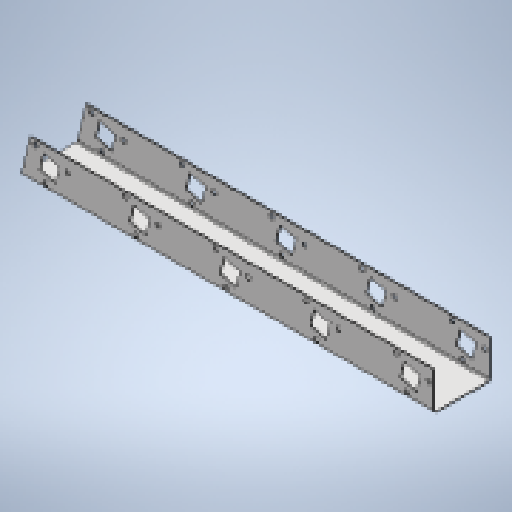
# Autodesk Inventor part: MNT-CDF-501 box
Saved by Autodesk Inventor 2025.1 (Build 291241020, 241B)
## iProperties
Created: 2025-01-13
Part Number: MNT-CDF-501 box
Material: Stainless Steel
Description: DIE16(5)|\ 90°|corrY -___°|X_____|bom___
Document SubType Name: Sheet Metal
Designer: user
Stock Number: МОО 305 шпангоут борт
Mass: 1762.25 g
Surface Area: 2283.33 cm^2
Volume: 220.281 cm^3
Density: 8 g/cm^3
Sheet Metal Rule: AISI304 2mm Die16
Sheet Metal Width: 0.000 mm
Sheet Metal Length: 0.000 mm
Sheet Metal Area: 0.000 mm^2
Appearance: Default
БОРТ_стрингер_3_высота: 63.000 mm
БОРТ_стрингер_4_высота: 48.000 mm
БОРТ_стрингер_5_высота: 54.000 mm
БОРТ_стрингер_6_высота: 81.000 mm
РЕБРА_глубина_паза: 28.000 mm
РЕБРА_вырез_на_полке: 5,000 mm
РЕБРА_полка: 20,000 mm
Author: user
Autodesk Inventor part; units mm, degrees
ref_plane "YZ Plane" through (0, 0, 0) normal (1, 0, 0) x (0, 1, 0)
ref_plane "XZ Plane" through (0, 0, 0) normal (0, 1, 0) x (-1, 0, 0)
ref_plane "XY Plane" through (0, 0, 0) normal (0, 0, 1) x (1, 0, 0)
sketch "Sketch1" plane through (0, 0, 0) normal (0, 0, 1) x (1, 0, 0)
  line L0 (0, -60) -> (870, -60)
  line L1 (870, -60) -> (870, 60)
  line L2 (870, 60) -> (0, 60)
  line L3 (0, 60) -> (0, -60)
  line L4 (0, -60) -> (870, 60) construction
  line L5 (870, -60) -> (0, 60) construction
  point P0 (0, 0)
  point P1 (0, 0)
  dimension "d154" = 870
  dimension "d155" = 120
  measures "d154" distance of L1.end L2.end
  measures "d155" distance of L0.end L1.end
extrude "Plate3" add sketch "Sketch1" along normal blind 2
sketch "Sketch7" plane through (870, -58, 0) normal (0, -1, 0) x (1, 0, 0)
  line L0 (-870, 0) -> (0, 0)
  line L1 (0, 0) -> (0, 80)
  line L2 (0, 80) -> (-870, 80)
  line L3 (-870, 80) -> (-870, 0)
  constraints: 6 end point, 1 horizontal, 1 perpendicular, 1 vertical
edge flange "Flange3" height 80 angle 90 thickness 2 bend radius 2.75 thickness toward (0, -1, 0) relief round relief width 2 relief depth 1 corner gap 2.75 corner form 0 edges at (435, -60, 2) (435, 60, 2) wall of the first edge with corners at (0, -58, 0) (870, -58, 0) (870, -58, 80) (0, -58, 80)
bend "Bend3"
corner "Corner3"
sketch "Sketch8" plane through (0, 0, 0) normal (0, 1, 0) x (-1, 0, 0)
  line L0 (0, 4.75) -> (0, 80) projected
  line L1 (-870, 80) -> (-870, 4.75) projected
  line L2 (-47.2535, 65.3406) -> (-81.2138, 56.8734)
  line L3 (-81.2138, 56.8734) -> (-72.7465, 22.913)
  line L4 (-72.7465, 22.913) -> (-38.7862, 31.3803)
  line L5 (-38.7862, 31.3803) -> (-47.2535, 65.3406)
  line L6 (-47.2535, 65.3406) -> (-72.7465, 22.913) construction
  line L7 (-81.2138, 56.8734) -> (-38.7862, 31.3803) construction
  circle A0 centre (-52.0166, 12.1071) radius 5.05
  circle A1 centre (-30.8781, 72) radius 5.05
  circle A2 centre (-98.7988, 55.0655) radius 5.05
  line L8 (-30.8781, 72) -> (-98.7988, 55.0655) construction
  line L9 (-98.7988, 55.0655) -> (-52.0166, 12.1071) construction
  line L10 (-52.0166, 12.1071) -> (-30.8781, 72) construction
  line L11 (-64.2336, 61.107) -> (-52.0166, 12.1071) construction
  line L12 (-870, 80) -> (0, 80) projected
  point P0 (0, 0)
  point P1 (-60, 44.1268)
  point P2 (0, 42.375)
  point P3 (-59.5888, 42.4775)
  dimension "d166" = 35
  dimension "d167" = 35
  dimension "d168" = 60
  dimension "d169" = 10.1
  dimension "d180" = 14
  dimension "d184" = 70
  dimension "d187" = 53
  dimension "d188" = 20
  dimension "d189" = 8
  constraints: 20 end point, 4 midpoint, 3 centre point, 3 parallel, 1 equal radius, 1 perpendicular, 1 point on line, 2 other
  measures "d166" distance of L4.end L3.end
  measures "d167" distance of L3.end L2.end
  measures "d168" distance from line of point (-60, 44.127) L0
  measures "d169" diameter of A0
  measures "d180" angle of L5 L0
  measures "d184" distance of L8.start L8.end
  measures "d187" distance from line of L9.end L8
  measures "d188" distance from line of L8 point (-60, 44.127)
  measures "d189" distance from line of L12 L8.start
extrude "Extrusion3" cut sketch "Sketch8" along normal through all both and the other way through all
pattern_linear "Rectangular Pattern4" count 5 spacing 190 along (1, 0, 0) of "Extrusion3"
sketch "Sketch9" plane through (0, 0, 0) normal (0, 1, 0) x (-1, 0, 0)
  line L0 (0, 80) -> (-870, 80) projected
  line L1 (0, 0) -> (-870, 0) projected
  line L2 (0, 0) -> (0, 80)
  line L3 (-870, 80) -> (0, 80) projected
  line L4 (-19.9462, 80) -> (0, 0)
  dimension "d181" = 14
  constraints: 4 end point, 1 perpendicular, 1 point on line
  measures "d181" angle of L2 L4
extrude "Extrusion4" cut sketch "Sketch9" along normal through all both and the other way through all
equation "\"БОРТ_стрингер_3_высота\" = 63"
equation "\"БОРТ_стрингер_4_высота\" = 48"
equation "\"БОРТ_стрингер_5_высота\" = 54"
equation "\"БОРТ_стрингер_6_высота\" = 81"
body "Solid2"
